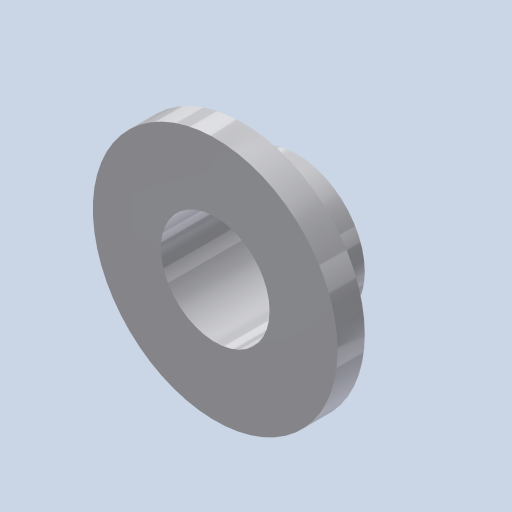
# Autodesk Inventor part: D4050-9120B
Saved by Autodesk Inventor 2023 (Build 270158000, 158)
## iProperties
Created: 2015-11-28
Part Number: D4050-9120B
Material: アセタール樹脂、白
Document SubType Name: Modeling
Designer: hiroaki
Density: 1.425 g/cm^3
Appearance: 積雪
Mass: 0.092893 g
Surface Area: 1.99491 cm^2
Volume: 0.065188 cm^3
Author: hiroaki
Autodesk Inventor part; units mm, degrees
ref_plane "YZ Plane" through (0, 0, 0) normal (1, 0, 0) x (0, 1, 0)
ref_plane "XZ Plane" through (0, 0, 0) normal (0, 1, 0) x (-1, 0, 0)
ref_plane "XY Plane" through (0, 0, 0) normal (0, 0, 1) x (1, 0, 0)
sketch "スケッチ1" plane through (0, 0, 0) normal (0, 0, 1) x (1, 0, 0)
  line L0 (2, 1.5) -> (2, -1.5)
  line L1 (2, -1.5) -> (4.5, -1.5)
  line L2 (4.5, -1.5) -> (4.5, -0.5)
  line L3 (4.5, -0.5) -> (2.5, -0.5)
  line L4 (2.5, -0.5) -> (2.5, 1.5)
  line L5 (2.5, 1.5) -> (2, 1.5)
  line L6 (0, 0) -> (0, 2.9634) construction
  point P0 (2, 0)
  dimension "d0" = 1
  dimension "d1" = 2
  dimension "d2" = 2.5
  dimension "d3" = 4.5
  dimension "d4" = 2
  constraints: 14 end point, 5 perpendicular, 2 vertical, 1 horizontal alignment, 1 midpoint
  measures "d0" distance of L1.end L2.end
  measures "d1" distance from line of L6.start L0
  measures "d2" distance between parallel lines of L6 L4
  measures "d3" distance between parallel lines of L6 L2
  measures "d4" distance of L3.end L4.end
revolve "回転1" add sketch "スケッチ1" angle 360 about axis through (0, 0, 0) along (0, 1, 0)
